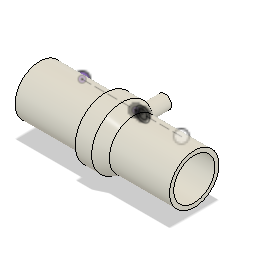
Oxygen Mixer V1 (Autodesk Fusion 360 design; units mm, degrees)
Autodesk Fusion 360 part; units mm, degrees
note: some values were not read from the file. Set by a fixed rule: which sketch regions a step uses.
sketch "Sketch7" plane through (0, 0, 0) normal (0, 1, 0) x (1, 0, 0)
  line L0 (15.0792, 9) -> (21.7323, 5.854)
  line L1 (21.7323, 5.854) -> (21.3049, 4.95)
  line L2 (21.3049, 4.95) -> (15.9121, 7.5)
  line L3 (15.9121, 7.5) -> (-9.9208, 7.5)
  line L4 (-9.9208, 7.5) -> (-9.9208, 9)
  line L5 (15.0792, 9) -> (15.0792, 10.0604)
  line L6 (15.0792, 10.0604) -> (19.8547, 10.0604)
  line L7 (19.8547, 10.0604) -> (24.7323, 7.7539)
  line L8 (24.7323, 7.7539) -> (24.7323, 4.95)
  line L9 (24.7323, 4.95) -> (25.7323, 4.95)
  line L10 (25.7323, 4.95) -> (25.7323, 7.5)
  line L11 (20.0792, 11.0604) -> (14.0792, 11.0604)
  line L12 (14.0792, 11.0604) -> (14.0792, 9)
  line L13 (24.4365, 9) -> (46.4365, 9)
  line L14 (46.4365, 9) -> (46.4365, 7.5)
  line L15 (46.4365, 7.5) -> (25.7323, 7.5)
  line L16 (-22.2609, 0) -> (38.4517, 0) construction
  line L17 (-9.9208, 9) -> (14.0792, 9)
  line L18 (24.4365, 9) -> (20.0792, 11.0604)
  line L19 (21.3049, 4.95) -> (24.7323, 4.95) construction
  line L20 (14.0792, 9) -> (15.0792, 9) construction
  dimension "d24" = 7.5
  dimension "d25" = 1.5
  dimension "d26" = 1
  dimension "d27" = 1
  dimension "d28" = 1
  dimension "d29" = 1
  dimension "d30" = 3
  dimension "d33" = 4.95
  dimension "d34" = 3
  dimension "d42" = 6
  dimension "d44" = 24
  dimension "d45" = 22
  constraint horizontal L17
  constraint perpendicular L0 L1
  constraint perpendicular L1 L2
  constraint perpendicular L5 L17
  constraint perpendicular L8 L9
  constraint perpendicular L9 L10
  constraint horizontal L11
  constraint perpendicular L12 L17
  constraint perpendicular L13 L14
  constraint perpendicular L14 L15
  constraint horizontal L16
  constraint coincident L16 origin
  constraint coincident L11.end L12.start
  constraint coincident L5.end L6.start
  constraint horizontal L6
  constraint vertical L4
  constraint equal L4 L14
  constraint horizontal L19
  constraint coincident L8.end L9.start
  constraint collinear L3 L15
  constraint parallel L0 L7
  constraint coincident L10.end L15.end
  constraint vertical L10
  constraint equal L1 L9
  constraint perpendicular L5 L20
  constraint coincident L0.start L5.start
  measures "d24" distance of L15 L16
  measures "d25" distance of L13.end L14.end
  measures "d26" distance of L8.end L9.end
  measures "d27" distance of L7 L18
  measures "d28" distance of L6 L11
  measures "d29" distance of L5 L12
  measures "d30" distance of L0.end L7
  measures "d33" distance of L1.end L16
  measures "d34" horizontal distance of L0.end L8.end
  measures "d42" distance of L11.start L11.end
  measures "d44" distance of L4.end L12.end
  measures "d45" distance of L13.start L13.end
revolve "Revolve1" add sketch "Sketch7" angle 360 about axis through (-22.2609, 0, 0) along (1, 0, 0) makes body 1 in component "Mixer"
ref_plane "WorkPlane5" through (17.1689, 0, -11.0604) normal (0, 0, -1) x (0, -1, 0)
sketch "Sketch9" plane through (-5.5333, 0, -11.0604) normal (0, 0, -1) x (1, 0, 0)
  circle A0 centre (22.1124, 0) radius 1.5
  circle A1 centre (22.1124, 0) radius 2.5
  line L0 (0, 0) -> (36.1934, 0) construction
  point P0 (19.6124, 0)
  point P1 (19.6124, 0)
  dimension "d36" = 3
  dimension "d37" = 1
  constraint concentric A0 A1
  constraint coincident L0.start origin
  constraint horizontal L0
  constraint coincident A0.centre L0
  constraint coincident L0 P1
  constraint coincident A1 P1
  constraint coincident P1 P0
  measures "d36" diameter of A0
  measures "d37" distance of A0 A1
extrude "Extrude2" cut sketch "Sketch9" along normal up to surface contours A0 end surface at (18.2628, -1.0017, -10.0104) on bodies 1 bodies 1 in component "Mixer"
extrude "Extrude2'" add sketch "Sketch9" along normal blind 8 separate body makes body 2
copy_body "CutPasteBodies2" bodies 2 removing the originals makes body 3 in component "Mixer"
component "Mixer" placed x (1, 0, 0) y (0, 1, 0) z (0, 0, 1) at (0, 0, 0)
